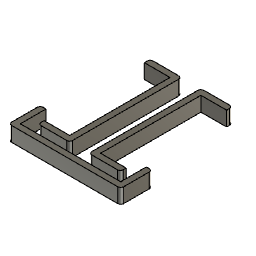
nato_strap_clasp (Autodesk Fusion 360 design; units mm, degrees)
Autodesk Fusion 360 part; units mm, degrees
sketch "Sketch1" plane through (0, 0, 0) normal (0, 0, 1) x (1, 0, 0)
  line L0 (0, 0) -> (21.844, 0)
  line L1 (21.844, 0) -> (21.844, 5.588)
  line L2 (21.844, 5.588) -> (23.114, 5.588)
  line L3 (23.114, 5.588) -> (23.114, -1.27)
  line L4 (0, 0) -> (0, 5.588)
  line L5 (0, 5.588) -> (-1.27, 5.588)
  line L6 (-1.27, 5.588) -> (-1.27, -1.27)
  line L7 (-1.27, -1.27) -> (23.114, -1.27)
  line L8 (21.844, 0) -> (19.5989, 2.2451) construction
  line L9 (21.844, 0) -> (25.019, 0) construction
  line L10 (21.7167, 5.588) -> (23.114, 5.588)
  line L11 (21.7167, 0.1273) -> (21.7167, 5.588)
  line L12 (0, 5.588) -> (-1.27, 5.588)
  line L13 (21.7167, 0.1273) -> (19.5989, 2.2451) construction
  line L14 (0, 0.1273) -> (21.7167, 0.1273)
  line L15 (0, 0) -> (0, 5.588)
  line L16 (-1.27, -1.27) -> (23.114, -1.27)
  line L17 (23.114, 5.588) -> (23.114, -1.27)
  line L18 (-1.27, 5.588) -> (-1.27, -1.27)
  line L19 (0, 5.588) -> (1.5875, 5.588) construction
  line L20 (1.9695, 0.1273) -> (1.9695, 1.9053) construction
  line L21 (1.9695, 1.9053) -> (8.8275, 1.9053)
  line L22 (8.8275, 1.9053) -> (8.8275, 26.2893)
  line L23 (8.8275, 26.2893) -> (1.9695, 26.2893)
  line L24 (1.9695, 1.9053) -> (1.9695, 3.1753)
  line L25 (1.9695, 3.1753) -> (7.5575, 3.1753)
  line L26 (1.9695, 26.2893) -> (1.9695, 25.0193)
  line L27 (1.9695, 25.0193) -> (7.5575, 25.0193)
  line L28 (7.5575, 3.1753) -> (7.5575, 25.0193)
  line L29 (13.0165, 26.2893) -> (19.8745, 26.2893)
  line L30 (19.8745, 26.2893) -> (19.8745, 25.0193)
  line L31 (19.8745, 25.0193) -> (14.2865, 25.0193)
  line L32 (14.2865, 3.1753) -> (14.2865, 25.0193)
  line L33 (13.0165, 1.9053) -> (13.0165, 26.2893)
  line L34 (19.8745, 1.9053) -> (13.0165, 1.9053)
  line L35 (19.8745, 3.1753) -> (14.2865, 3.1753)
  line L36 (19.8745, 1.9053) -> (19.8745, 3.1753)
  point P0 (0, 0.1273)
  dimension "d15" = 1.5875
  dimension "d16" = 1.778
  dimension "d17" = 6.858
  dimension "d18" = 24.384
  dimension "d19" = 6.858
  dimension "d20" = 1.27
  dimension "d21" = 5.588
  dimension "d22" = 1.27
  dimension "d23" = 5.588
  constraint coincident L0.start L4.start
  constraint horizontal L0
  constraint perpendicular L0 L1
  constraint perpendicular L1 L2
  constraint perpendicular L2 L3
  constraint horizontal L9
  constraint coincident P0 L14.start
  constraint horizontal L14
  constraint perpendicular L11 L14
  constraint perpendicular L10 L11
  constraint perpendicular L10 L17
  constraint perpendicular L4 L19
  constraint coincident L14 L20.start
  constraint perpendicular L0 L20
  constraint perpendicular L20 L21
  constraint perpendicular L21 L22
  constraint perpendicular L22 L23
  constraint perpendicular L21 L24
  constraint perpendicular L24 L25
  constraint perpendicular L23 L26
  constraint perpendicular L26 L27
  measures "d15" distance of L4.end L19.end
  measures "d16" distance of L20.start L20.end
  measures "d17" distance of L20.end L21.end
  measures "d18" distance of L21.end L22.end
  measures "d19" distance of L22.end L23.end
  measures "d20" distance of L20.end L24.end
  measures "d21" distance of L24.end L25.end
  measures "d22" distance of L23.end L26.end
  measures "d23" distance of L26.end L27.end
extrude "Extrude1" add sketch "Sketch1" along normal blind 3.175 contours L0 L1 L2 L3 L4 L5 L6 L7 L10 L12 L15 L16 L17 L18 | L21 L22 L23 L24 L25 L26 L27 L28 | L29 L30 L31 L32 L33 L34 L35 L36 makes body 1 at (14.986, -1.27, 2.1167) makes body 2 at (8.8275, 18.1613, 2.1167) makes body 3 at (13.0165, 18.1613, 2.1167)
fillet "Fillet1" radius 0.635 8 edges at (-1.27, -1.27, 1.5875) (23.114, -1.27, 1.5875) (-1.27, 5.588, 1.5875) (23.114, 5.588, 1.5875) (1.9695, 1.9053, 1.5875) (8.8275, 1.9053, 1.5875) (8.8275, 26.2893, 1.5875) (1.9695, 26.2893, 1.5875) on bodies 1 2 3
fillet "Fillet1" radius 0.635 4 edges at (19.8745, 1.9053, 1.5875) (13.0165, 1.9053, 1.5875) (13.0165, 26.2893, 1.5875) (19.8745, 26.2893, 1.5875) on bodies 1 2 3
